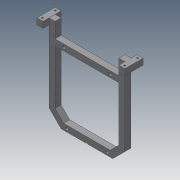
# Autodesk Inventor part: Base
Saved by Autodesk Inventor 2014 SP1 (Build 180222100, 222)
## iProperties
Created: 2013-12-26
Part Number: Base
Material: Generic
Document SubType Name: Modeling
Designer: tom
Density: 1 g/cm^3
Appearance: Default
Author: tom
Autodesk Inventor part; units mm, degrees
ref_plane "YZ Plane" through (0, 0, 0) normal (1, 0, 0) x (0, 1, 0)
ref_plane "XZ Plane" through (0, 0, 0) normal (0, 1, 0) x (-1, 0, 0)
ref_plane "XY Plane" through (0, 0, 0) normal (0, 0, 1) x (1, 0, 0)
sketch "Sketch1" plane through (0, 0, 0) normal (0, 0, 1) x (1, 0, 0)
  line L0 (-73.0208, 6.3503) -> (73.0288, 6.3503) construction
  line L1 (73.0288, 6.3503) -> (73.0288, 150.3683) construction
  line L2 (73.0288, 150.3683) -> (-73.0208, 150.3683) construction
  line L3 (-73.0208, 150.3683) -> (-73.0208, 6.3503) construction
  line L4 (-79.3708, 156.7183) -> (79.3788, 156.7183) construction
  line L5 (79.3788, 188.4683) -> (79.3788, 0.0003) construction
  line L6 (79.3788, 0.0003) -> (-79.3708, 0.0003) construction
  line L7 (-79.3708, 0.0003) -> (-79.3708, 156.7183) construction
  line L8 (-66.6708, 144.0183) -> (66.6788, 144.0183) construction
  line L9 (66.6788, 144.0183) -> (66.6788, 12.7003) construction
  line L10 (66.6788, 12.7003) -> (-66.6708, 12.7003) construction
  line L11 (-66.6708, 12.7003) -> (-66.6708, 156.7183) construction
  line L12 (79.3788, 156.7183) -> (66.6788, 144.0183) construction
  line L13 (-79.3708, 156.7183) -> (-66.6708, 144.0183) construction
  line L14 (-53.9708, 131.3183) -> (53.9788, 131.3183) construction
  line L15 (53.9788, 131.3183) -> (53.9788, 25.4003) construction
  line L16 (53.9788, 25.4003) -> (-53.9708, 25.4003) construction
  line L17 (-53.9708, 25.4003) -> (-53.9708, 131.3183) construction
  line L18 (-53.9708, 156.7183) -> (-79.3708, 131.3183) construction
  line L19 (-48.7103, 144.0183) -> (-66.6708, 126.0578) construction
  line L20 (0.004, 131.3183) -> (0.004, 156.7183) construction
  line L21 (-53.9708, 78.3593) -> (-79.3708, 78.3593) construction
  line L22 (-66.6708, 156.7183) -> (66.6788, 156.7183)
  line L23 (-79.3708, 25.4003) -> (-53.9708, 0.0003)
  line L24 (-53.9708, 0.0003) -> (53.9788, 0.0003)
  line L25 (-66.6708, 30.6608) -> (-48.7103, 12.7003)
  line L26 (-48.7103, 12.7003) -> (0.0038, 12.7003)
  line L27 (48.7183, 12.7003) -> (0.0038, 12.7003)
  line L28 (79.3788, 25.4003) -> (53.9788, 0.0003)
  line L29 (66.6788, 144.0183) -> (66.6788, 30.6608)
  line L30 (66.6788, 30.6608) -> (48.7183, 12.7003)
  line L31 (79.3788, 188.4683) -> (79.3788, 25.4003)
  line L32 (-66.6708, 144.0183) -> (66.6788, 144.0183)
  line L33 (-66.6708, 144.0183) -> (-66.6708, 30.6608)
  line L34 (-79.3708, 25.4003) -> (-79.3708, 188.4683)
  line L35 (-66.6708, 156.7183) -> (-66.6708, 188.4683)
  line L36 (-66.6708, 188.4683) -> (-79.3708, 188.4683)
  line L37 (66.6788, 156.7183) -> (66.6788, 188.4683)
  line L38 (66.6788, 188.4683) -> (79.3788, 188.4683)
  line L39 (-48.7103, 156.7183) -> (-48.7103, 0.0003) construction
  line L40 (48.7183, 156.7183) -> (48.7183, 0.0003) construction
  circle A0 centre (-42.3603, 6.3503) radius 3.175
  circle A1 centre (42.3683, 6.3503) radius 3.175
  circle A2 centre (-48.7103, 150.3683) radius 3.175
  circle A3 centre (48.7183, 150.3683) radius 3.175
  point P0 (79.3788, 131.3183)
  dimension "d1" = 144.018
  dimension "d2" = 6.35
  dimension "d3" = 6.35
  dimension "d4" = 12.7
  dimension "d5" = 12.7
  dimension "d22" = 6.35
  dimension "d23" = 6.35
  dimension "d24" = 6.35
  dimension "d25" = 6.35
  dimension "d26" = 6.35
  dimension "d27" = 6.35
  constraints: 82 end point, 27 point on line, 14 perpendicular, 9 symmetric about line, 6 midpoint, 6 parallel, 4 centre point, 1 collinear, 1 horizontal, 6 other
  measures "d1" distance of L0.end L1.end
  measures "d2" distance between parallel lines of L2 L4
  measures "d3" distance between parallel lines of L8 L2
  measures "d4" distance between parallel lines of L8 L14
  measures "d5" distance between parallel lines of L18 L19
  measures "d22" diameter of A0
  measures "d23" distance from line of L39 A0.centre
  measures "d24" diameter of A1
  measures "d25" distance from line of L40 A1.centre
  measures "d26" diameter of A2
  measures "d27" diameter of A3
extrude "Extrusion1" add sketch "Sketch1" against normal blind 12.7
sketch "Sketch4" plane through (0, 0, -12.7) normal (0, 0, -1) x (-1, 0, 0)
  line L0 (-79.3788, 188.4683) -> (-79.3788, 25.4003) projected
  line L1 (-53.9788, 0.0003) -> (53.9708, 0.0003) projected
  line L2 (-79.3788, 188.4683) -> (-92.0788, 188.4683)
  line L3 (-92.0788, 188.4683) -> (-92.0788, 175.7683)
  line L4 (-92.0788, 175.7683) -> (-79.3788, 175.7683)
  line L5 (-79.3788, 175.7683) -> (-79.3788, 189.4306)
  point P0 (0, 0)
  dimension "d15" = 12.7
  dimension "d16" = 12.7
  constraints: 8 end point, 2 parallel, 2 perpendicular, 1 point on line
  measures "d15" distance of L0.start L2.end
  measures "d16" distance of L2.end L3.end
extrude "Extrusion4" add sketch "Sketch4" along normal blind 12.7 and the other way blind 25.4
mirror "Mirror1" about plane through (0, 0, 0) normal (1, 0, 0) of "Extrusion4"
sketch "Sketch6" plane through (79.3788, 175.7683, -25.4) normal (0, -1, 0) x (1, 0, 0)
  circle A0 centre (6.7505, 32.5247) radius 1.7526
  circle A1 centre (6.7505, 5.5753) radius 1.7526
  line L0 (0, 12.7) -> (0, 25.4) projected
  line L1 (12.7, 38.1) -> (12.7, 0) projected
  line L2 (12.7, 19.05) -> (0, 19.05) construction
  point P0 (-79.3788, 25.4)
  dimension "d30" = 13.4747
  dimension "d31" = 26.9494
  constraints: 2 centre point, 2 end point, 2 midpoint
  measures "d30" distance from line of L2 A0.centre
  measures "d31" distance of A1.centre A0.centre
extrude "Extrusion5" cut sketch "Sketch6" against normal blind 12.7
mirror "Mirror2" about plane through (0, 0, 0) normal (1, 0, 0) of "Extrusion5"
body "Solid1"
